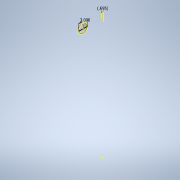
# Autodesk Inventor part: end cap B
Saved by Autodesk Inventor 2021 (Build 250183000, 183)
## iProperties
Created: 2021-08-25
Part Number: end cap B
Material: Generic
Document SubType Name: Modeling
Designer: newic
Density: 1 g/cm^3
Appearance: Default
Author: newic
Autodesk Inventor part; units mm, degrees
ref_plane "XZ Plane" through (0, 0, 0) normal (0, 1, 0) x (-1, 0, 0)
ref_plane "XY Plane" through (0, 0, 0) normal (0, 0, 1) x (1, 0, 0)
sketch "Sketch1" plane through (0, 0, 0) normal (1, 0, 0) x (0, 1, 0)
  line L0 (920.75, 0) -> (0, 0)
  line L1 (0, 0) -> (920.75, 0)
  line L2 (-297.6389, 409.8513) -> (2710.7909, 409.8513) construction
  line L3 (2710.7909, 409.8513) -> (2710.7909, -1716.9746) construction
  line L4 (2710.7909, -1716.9746) -> (-297.6389, -1716.9746) construction
  line L5 (-297.6389, -1716.9746) -> (-297.6389, 409.8513) construction
  line L6 (0, 0) -> (920.75, 0)
  line L7 (920.75, 0) -> (920.75, 100.33)
  line L8 (0, 100.33) -> (920.75, 100.33)
  line L9 (0, 0) -> (0, 100.33)
  line L10 (0, 100.33) -> (0, 120.65)
  line L11 (0, 120.65) -> (920.75, 120.65)
  line L12 (920.75, 120.65) -> (920.75, 100.33)
  line L13 (0, 120.65) -> (0, 196.85)
  line L14 (477.9962, 0) -> (477.9962, -13.97)
  line L15 (477.9962, -13.97) -> (434.8162, -13.97)
  line L16 (434.8162, -13.97) -> (434.8162, 0)
  line L17 (133.294, 0) -> (133.294, -13.97)
  line L18 (133.294, -13.97) -> (90.114, -13.97)
  line L19 (90.114, -13.97) -> (90.114, 0)
  line L20 (769.0257, 0) -> (769.0257, -13.97)
  line L21 (769.0257, -13.97) -> (812.2057, -13.97)
  line L22 (812.2057, -13.97) -> (812.2057, 0)
  line L23 (434.8162, -13.97) -> (477.9962, -13.97)
  line L24 (769.0257, -13.97) -> (812.2057, -13.97)
  line L25 (90.114, -13.97) -> (133.294, -13.97)
  line L26 (90.114, -13.97) -> (111.704, -13.97)
  line L27 (111.704, -13.97) -> (100.909, -13.97)
  line L28 (100.909, -13.97) -> (122.499, -13.97)
  line L29 (122.499, -13.97) -> (122.499, -33.02)
  line L30 (122.499, -33.02) -> (100.909, -33.02)
  line L31 (100.909, -33.02) -> (100.909, -13.97)
  line L32 (434.8162, -13.97) -> (456.4062, -13.97)
  line L33 (456.4062, -13.97) -> (445.6112, -13.97)
  line L34 (445.6112, -13.97) -> (467.2012, -13.97)
  line L35 (467.2012, -13.97) -> (467.2012, -33.02)
  line L36 (467.2012, -33.02) -> (445.6112, -33.02)
  line L37 (445.6112, -33.02) -> (445.6112, -13.97)
  line L38 (769.0257, -13.97) -> (790.6157, -13.97)
  line L39 (790.6157, -13.97) -> (779.8207, -13.97)
  line L40 (779.8207, -13.97) -> (801.4107, -13.97)
  line L41 (801.4107, -13.97) -> (801.4107, -33.02)
  line L42 (801.4107, -33.02) -> (779.8207, -33.02)
  line L43 (779.8207, -33.02) -> (779.8207, -13.97)
  line L44 (434.8162, 0) -> (413.2262, 0)
  line L45 (413.2262, 0) -> (413.2262, -11.43)
  line L46 (413.2262, -11.43) -> (371.9512, -11.43)
  line L47 (371.9512, -11.43) -> (371.9512, 64.77)
  arc A0 (413.2262, 72.0379) -> (371.9512, 72.0379) centre (392.5887, 68.404) ccw
  line L48 (413.2262, 0) -> (413.2262, 64.77)
  line L49 (371.9512, 64.77) -> (371.9512, 72.0379)
  line L50 (413.2262, 64.77) -> (413.2262, 72.0379)
  line L51 (434.8162, -13.97) -> (434.8162, 202.565)
  line L52 (477.9962, -13.97) -> (477.9962, 202.565)
  line L53 (769.0257, -13.97) -> (769.0257, 202.565)
  line L54 (812.2057, -13.97) -> (812.2057, 202.565)
  line L55 (812.2057, 202.565) -> (769.0257, 202.565)
  line L56 (477.9962, 202.565) -> (434.8162, 202.565)
  line L57 (133.294, -13.97) -> (133.294, 182.245)
  line L58 (90.114, -13.97) -> (90.114, 182.245)
  line L59 (90.114, 182.245) -> (133.294, 182.245)
  line L60 (67.3834, 182.245) -> (164.6776, 182.245)
  line L61 (413.2262, 202.565) -> (508.4774, 202.565)
  line L62 (745.5808, 202.565) -> (847.3717, 202.565)
  line L63 (67.3834, 161.925) -> (164.6776, 161.925)
  line L64 (413.2262, 182.245) -> (508.4774, 182.245)
  line L65 (745.5808, 182.245) -> (847.3717, 182.245)
  line L66 (133.294, -13.97) -> (133.294, 78.74)
  line L67 (133.294, 78.74) -> (434.8162, 78.74)
  line L68 (133.294, -13.97) -> (133.294, 26.67)
  line L69 (133.294, 26.67) -> (371.9512, 26.67)
  line L70 (133.294, 26.67) -> (298.394, 26.67)
  line L71 (298.394, 26.67) -> (317.7759, 78.74)
  line L72 (133.294, 78.74) -> (133.294, 59.055)
  line L73 (133.294, 59.055) -> (310.4486, 59.055)
  line L74 (905.6652, 120.65) -> (905.6652, 196.85)
  line L75 (905.6652, 120.65) -> (936.6408, 153.8672)
  line L76 (905.6652, 196.85) -> (940.9781, 158.9816)
  line L77 (905.6652, 158.75) -> (923.3216, 158.75)
  line L78 (923.3216, 158.75) -> (923.3216, 177.9158)
  line L79 (923.3216, 158.75) -> (923.3216, 139.5842)
  circle A1 centre (1042.6056, 173.924) radius 19.1643
  dimension "d0" = 920.75
  dimension "d1" = 20.32
  dimension "d2" = 76.2
  dimension "d3" = 13.97
  dimension "d4" = 43.18
  dimension "d5" = 13.97
  dimension "d6" = 43.18
  dimension "d7" = 13.97
  dimension "d8" = 13.97
  dimension "d9" = 43.18
  dimension "d10" = 21.59
  dimension "d11" = 19.05
  dimension "d12" = 21.59
  dimension "d13" = 19.05
  dimension "d14" = 21.59
  dimension "d15" = 19.05
  dimension "d16" = 21.59
  dimension "d17" = 11.43
  dimension "d18" = 41.275
  dimension "d19" = 76.2
  dimension "d20" = 20.955
  dimension "d21" = 216.535
  dimension "d22" = 216.535
  dimension "d23" = 216.535
  dimension "d24" = 216.535
  dimension "d25" = 196.215
  dimension "d26" = 20.32
  dimension "d27" = 20.32
  dimension "d28" = 20.32
  dimension "d29" = 92.71
  dimension "d30" = 40.64
  dimension "d31" = 165.1
  dimension "d32" = 19.685
  dimension "d35" = 76.2
  dimension "d36" = 43
  dimension "d37" = 43
  dimension "d38" = 38.3316
  dimension "d39" = 38.3286
  constraints: 150 end point, 14 perpendicular, 13 horizontal, 13 point on line, 12 vertical, 10 equal length, 9 midpoint, 2 centre point, 2 point on circle, 12 other
  measures "d0" distance of L0.start L0.end
  measures "d1" distance of L8.start L10.end
  measures "d2" distance of L10.end L13.end
  measures "d3" distance of L14.start L14.end
  measures "d4" distance of L14.end L15.end
  measures "d5" distance of L17.start L17.end
  measures "d6" distance of L17.end L18.end
  measures "d7" distance of L18.end L19.end
  measures "d8" distance of L20.start L20.end
  measures "d9" distance of L20.end L21.end
  measures "d10" distance of L29.end L30.end
  measures "d11" distance of L28.end L29.end
  measures "d12" distance of L35.end L36.end
  measures "d13" distance of L34.end L35.end
  measures "d14" distance of L41.end L42.end
  measures "d15" distance of L40.end L41.end
  measures "d16" distance of L16.end L44.end
  measures "d17" distance of L44.end L45.end
  measures "d18" distance of L45.end L46.end
  measures "d19" distance of L46.end L47.end
  measures "d20" radius of A0
  measures "d21" distance of L15.end L51.end
  measures "d22" distance of L23.end L52.end
  measures "d23" distance of L20.end L53.end
  measures "d24" distance of L24.end L54.end
  measures "d25" distance of L25.end L57.end
  measures "d26" distance between parallel lines of L60 L63
  measures "d27" distance between parallel lines of L61 L64
  measures "d28" distance between parallel lines of L62 L65
  measures "d29" distance of L25.end L66.end
  measures "d30" distance of L25.end L68.end
  measures "d31" distance of L68.end L70.end
  measures "d32" distance of L66.end L72.end
  measures "d35" distance of L74.start L74.end
  measures "d36" angle of L76 L74
  measures "d37" angle of L75 L74
  measures "d38" distance of L78.end L79.end
  measures "d39" diameter of A1
ref_plane "Work Plane1" through (17.653, 0, 0) normal (1, 0, 0) x (0, 1, 0)
sketch "Sketch2" plane through (17.653, 0, 0) normal (1, 0, 0) x (0, 1, 0)
  circle A0 centre (1042.6056, 173.924) radius 19.1643 projected
  circle A1 centre (1042.6056, 173.924) radius 38.1
  point P0 (0, 0)
  dimension "d41" = 76.2
  constraints: 1 centre point, 1 coincident
  measures "d41" diameter of A1
loft "Loft1" add profiles "Sketch2", "Sketch1" contours A0 | A1 / A1
shell "Shell1" thickness 2.54 removed faces 1 at (17.653, 1030.2684, 183.3553)
sketch "Sketch3" plane through (17.653, 1042.6056, 173.924) normal (1, 0, 0) x (0, 0, -1)
  circle A0 centre (0, 0) radius 38.1 projected
  line L0 (-38.1, 0) -> (38.1, 0)
  point P0 (173.924, -1042.6056)
  dimension "d47" = 76.2
  constraints: 2 end point, 2 point on circle, 1 horizontal
  measures "d47" distance of L0.end L0.start
sketch "Sketch4" plane through (0, 0, 0) normal (0, 0, 1) x (1, 0, 0)
  line L0 (17.653, 1080.7056) -> (17.653, 1004.5056) projected
  line L1 (0, 1023.4413) -> (0, 1061.7699) projected
  point P0 (0, 0)
  dimension "d48" = 17.653
  measures "d48" distance between parallel lines of L0 L1
body "Solid1"
